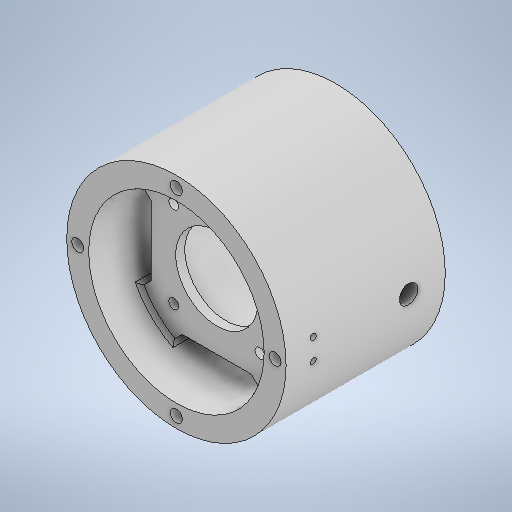
# Autodesk Inventor part: j1 57 mount
Saved by Autodesk Inventor 2025 (Build 290162000, 162)
## iProperties
Created: 2025-07-04
Part Number: j1 57 mount
Material: 一般
Document SubType Name: Modeling
Designer: gavin
Density: 1 g/cm^3
Appearance: 預設
Author: gavin
Autodesk Inventor part; units mm, degrees
ref_plane "XZ Plane" through (0, 0, 0) normal (0, 1, 0) x (-1, 0, 0)
ref_plane "XY Plane" through (0, 0, 0) normal (0, 0, 1) x (1, 0, 0)
sketch "草圖1" plane through (0, 0, 0) normal (0, 0, 1) x (1, 0, 0)
  circle A0 centre (0, 0) radius 60
  circle A1 centre (0, 0) radius 48
  dimension "d0" = 120
  dimension "d1" = 96
  constraints: 2 centre point, 2 coincident
  measures "d0" diameter of A0
  measures "d1" diameter of A1
extrude "擠出1" add sketch "草圖1" along normal blind 27.1 and the other way blind 60
sketch "草圖2" plane through (0, 0, 27.1) normal (0, 0, 1) x (1, 0, 0)
  circle A0 centre (0, 0) radius 54 construction
  circle A1 centre (0, 54) radius 3.275
  circle A2 centre (-54, 0) radius 3.275
  circle A3 centre (0, -54) radius 3.275
  circle A4 centre (54, 0) radius 3.275
  dimension "d6" = 108
  dimension "d7" = 6.55
  dimension "d10" = 360
  constraints: 4 centre point, 1 coincident, 1 vertical alignment, 11 other
  measures "d7" diameter of A1
extrude "擠出2" cut sketch "草圖2" against normal blind 20
ref_plane "工作平面1" through (0, 0, 0) normal (0, 0, 1) x (1, 0, 0)
sketch "草圖3" plane through (0, 0, 0) normal (0, 0, 1) x (1, 0, 0)
  circle A0 centre (-23.57, 23.57) radius 2.3
  circle A1 centre (23.57, 23.57) radius 2.3
  circle A2 centre (23.57, -23.57) radius 2.3
  circle A3 centre (-23.57, -23.57) radius 2.3
  circle A4 centre (-23.57, 23.57) radius 2.7
  circle A5 centre (23.57, 23.57) radius 2.7
  circle A6 centre (23.57, -23.57) radius 2.7
  circle A7 centre (-23.57, -23.57) radius 2.7
  circle A8 centre (0, 0) radius 22.5
  line L0 (-21.94355, 4.972987) -> (-41.348635, 24.378072)
  circle A9 centre (0, 0) radius 48
  line L1 (-24.378072, 41.348635) -> (-4.972987, 21.94355)
  line L2 (-23.57, 23.57) -> (0, 0) construction
  circle A10 centre (0, 0) radius 40.5
  line L3 (-41.348635, -24.378072) -> (-21.94355, -4.972987)
  line L4 (-4.972987, -21.94355) -> (-24.378072, -41.348635)
  line L5 (24.378072, -41.348635) -> (4.972987, -21.94355)
  line L6 (21.94355, -4.972987) -> (41.348635, -24.378072)
  line L7 (41.348635, 24.378072) -> (21.94355, 4.972987)
  line L8 (4.972987, 21.94355) -> (24.378072, 41.348635)
  point P0 (-18.866592, 35.837155)
  point P1 (-35.837155, 18.866592)
  point P2 (-35.837155, -18.866592)
  point P3 (-24.378072, -41.348635)
  point P4 (-18.866592, -35.837155)
  point P5 (18.866592, -35.837155)
  point P6 (24.378072, -41.348635)
  point P7 (41.348635, -24.378072)
  point P8 (35.837155, -18.866592)
  point P9 (35.837155, 18.866592)
  point P10 (41.348635, 24.378072)
  point P11 (24.378072, 41.348635)
  point P12 (18.866592, 35.837155)
  dimension "d14" = 5.4
  dimension "d15" = 5.4
  dimension "d16" = 5.4
  dimension "d17" = 5.4
  dimension "d18" = 45
  dimension "d19" = 24
  dimension "d20" = 12
  dimension "d21" = 18
  dimension "d24" = 360
  constraints: 18 end point, 6 centre point, 4 point on circle, 2 coincident, 2 parallel, 25 other
  measures "d14" diameter of A4
  measures "d15" diameter of A5
  measures "d16" diameter of A6
  measures "d17" diameter of A7
  measures "d18" diameter of A8
  measures "d19" distance between parallel lines of L1 L0
  measures "d20" distance from line of A0.centre L1
  measures "d21" radial gap between concentric circles of A8 A10
extrude "擠出3" add sketch "草圖3" along normal blind 5 contours A8 L7 A10 L6 | A8 L8 A10 L7 | L6 A10 L5 A8 | A8 L1 A10 L8 | A10 L8 A9 L7 | L5 A10 L4 A8 | L6 A9 L5 A10 | A8 L0 A10 L1 | L4 A10 L3 A8 | A8 L3 A10 L0 | A10 L0 A9 L1 | L4 A9 L3 A10
fillet "圓角1" radius 2 16 edges at (-33.9411, 33.9411, 5) (-41.3486, 24.3781, 2.5) (33.9411, 33.9411, 5) (41.3486, 24.3781, 2.5) (41.3486, -24.3781, 2.5) (33.9411, -33.9411, 5) (-33.9411, -33.9411, 5) (-41.3486, -24.3781, 2.5) (24.3781, 41.3486, 2.5) (24.3781, -41.3486, 2.5) (-24.3781, 41.3486, 2.5) (-24.3781, -41.3486, 2.5) (33.9411, -33.9411, 0) (-33.9411, -33.9411, 0) (-33.9411, 33.9411, 0) (33.9411, 33.9411, 0)
sketch "草圖4" plane through (0, 0, -60) normal (0, 0, -1) x (-1, 0, 0)
  circle A0 centre (0, 0) radius 54 construction
  circle A1 centre (0, -54) radius 3.275
  circle A2 centre (0, -54) radius 3.275
  circle A3 centre (46.765372, -27) radius 3.275
  circle A4 centre (46.765372, 27) radius 3.275
  circle A5 centre (0, 54) radius 3.275
  circle A6 centre (-46.765372, 27) radius 3.275
  circle A7 centre (-46.765372, -27) radius 3.275
  dimension "d29" = 108
  dimension "d32" = 360
  constraints: 7 centre point, 2 coincident, 1 concentric, 13 other
  measures "d29" diameter of A0
extrude "擠出4" cut sketch "草圖4" against normal blind 20
ref_plane "工作平面2" through (28.2, -16.65, -54) normal (1, 0, 0) x (0, 1, 0)
sketch "草圖5" plane through (28.2, -16.65, -54) normal (1, 0, 0) x (0, 1, 0)
  circle A0 centre (16.65, 14) radius 5
  line L0 (-43.35, -6) -> (76.65, -6) projected
  point P0 (16.65, 54)
  dimension "d36" = 10
  dimension "d37" = 20
  constraints: 1 centre point
  measures "d36" diameter of A0
  measures "d37" distance from line of L0 A0.centre
extrude "擠出5" cut sketch "草圖5" along normal through all
ref_plane "工作平面3" through (48, 0, 0) normal (1, 0, 0) x (0, 1, 0)
sketch "草圖7" plane through (48, 0, 0) normal (1, 0, 0) x (0, 1, 0)
  line L0 (9, 15.1) -> (-9, 15.1)
  line L1 (-9, 15.1) -> (-9, 8.85)
  line L2 (-9, 8.85) -> (9, 8.85)
  line L3 (9, 8.85) -> (9, 15.1)
  line L4 (-48, 27.1) -> (48, 27.1) projected
  point P0 (0, 0)
  dimension "d45" = 18
  dimension "d46" = 9
  dimension "d47" = 6.25
  dimension "d48" = 12
  constraints: 8 end point, 2 parallel, 1 horizontal, 1 perpendicular
  measures "d45" distance of L2.end L1.end
  measures "d46" distance from line of point (0, 0) L1
  measures "d47" distance of L2.end L0.start
  measures "d48" distance between parallel lines of L0 L4
extrude "擠出6" add sketch "草圖7" against normal blind 0.85
sketch "草圖8" plane through (47.15, 0, 0) normal (-1, 0, 0) x (0, 0, 1)
  line L0 (15.1, -8.993192) -> (8.85, -8.993192)
  line L1 (15.1, -8.993192) -> (15.1, 8.993192)
  line L2 (8.85, 8.993192) -> (15.1, 8.993192)
  line L3 (8.85, 8.993192) -> (8.85, -8.993192)
  line L4 (15.1, 0) -> (8.85, 0)
  circle A0 centre (11.975, 5.75) radius 1.6
  circle A1 centre (11.975, -5.75) radius 1.6
  point P0 (0, 0)
  point P1 (11.975, 8.993192)
  dimension "d52" = 3.2
  dimension "d53" = 5.75
  constraints: 3 midpoint, 2 centre point, 2 end point, 1 symmetric about line, 1 vertical alignment, 1 other
  measures "d52" diameter of A0
  measures "d53" distance from line of L4 A0.centre
extrude "擠出7" cut sketch "草圖8" against normal through all contours A0 | A1
sketch "草圖9" plane through (0, 0, 5) normal (0, 0, 1) x (1, 0, 0)
  arc A0 (-39.928224, -22.841561) -> (-22.841561, -39.928224) centre (0, 0) ccw
  arc A1 (-22.498585, -39.469148) -> (-22.841561, -39.928224) centre (-21.084372, -40.883362) ccw
  line L0 (-22.498585, -39.469148) -> (-18.866592, -35.837155)
  arc A2 (-18.866592, -35.837155) -> (18.866592, -35.837155) centre (0, 0) ccw
  line L1 (18.866592, -35.837155) -> (22.498585, -39.469148)
  arc A3 (22.841561, -39.928224) -> (22.498585, -39.469148) centre (21.084372, -40.883362) ccw
  arc A4 (22.841561, -39.928224) -> (39.928224, -22.841561) centre (0, 0) ccw
  arc A5 (39.469148, -22.498585) -> (39.928224, -22.841561) centre (40.883362, -21.084372) ccw
  line L2 (39.469148, -22.498585) -> (35.837155, -18.866592)
  arc A6 (35.837155, -18.866592) -> (35.837155, 18.866592) centre (0, 0) ccw
  line L3 (35.837155, 18.866592) -> (39.469148, 22.498585)
  arc A7 (39.928224, 22.841561) -> (39.469148, 22.498585) centre (40.883362, 21.084372) ccw
  arc A8 (39.928224, 22.841561) -> (22.841561, 39.928224) centre (0, 0) ccw
  arc A9 (22.498585, 39.469148) -> (22.841561, 39.928224) centre (21.084372, 40.883362) ccw
  line L4 (22.498585, 39.469148) -> (18.866592, 35.837155)
  arc A10 (18.866592, 35.837155) -> (-18.866592, 35.837155) centre (0, 0) ccw
  line L5 (-18.866592, 35.837155) -> (-22.498585, 39.469148)
  arc A11 (-22.841561, 39.928224) -> (-22.498585, 39.469148) centre (-21.084372, 40.883362) ccw
  arc A12 (-22.841561, 39.928224) -> (-39.928224, 22.841561) centre (0, 0) ccw
  arc A13 (-39.469148, 22.498585) -> (-39.928224, 22.841561) centre (-40.883362, 21.084372) ccw
  line L6 (-39.469148, 22.498585) -> (-35.837155, 18.866592)
  arc A14 (-35.837155, 18.866592) -> (-35.837155, -18.866592) centre (0, 0) ccw
  line L7 (-35.837155, -18.866592) -> (-39.469148, -22.498585)
  arc A15 (-39.928224, -22.841561) -> (-39.469148, -22.498585) centre (-40.883362, -21.084372) ccw
  circle A16 centre (23.57, -23.57) radius 2.7
  circle A17 centre (23.57, 23.57) radius 2.7
  circle A18 centre (-23.57, 23.57) radius 2.7
  circle A19 centre (-23.57, -23.57) radius 2.7
  circle A20 centre (0, 0) radius 22.5
  line L8 (18.866592, -35.837155) -> (-18.866592, -35.837155)
  line L9 (35.837155, 18.866592) -> (35.837155, -18.866592)
  line L10 (-18.866592, 35.837155) -> (18.866592, 35.837155)
  line L11 (-35.837155, -18.866592) -> (-35.837155, 18.866592)
  point P0 (35.837155, 18.866592)
  point P1 (-18.866592, 35.837155)
  point P2 (-35.837155, -18.866592)
  dimension "d58" = 360
  constraints: 8 end point, 1 horizontal, 13 other
extrude "擠出8" cut sketch "草圖9" against normal up to surface (5 mm away) contours A14 L11 | L8 A2 | A10 L10 | L9 A6
equation "\"d20\" = 0.5 * d19"
equation "\"d46\" = 0.5 * d45"
